Autodesk Fusion 360 part; units mm, degrees
(part 3 of 3)
sketch "Sketch3" plane through (0, 0, 2) normal (0, 0, 1) x (-1, 0, 0)
  line L0 (-24.5, 34.5) -> (-24.5, 36.0424)
  line L1 (-24.5, 36.0424) -> (-65.0462, 36.0424)
  arc A0 (-65.0462, 36.0424) -> (-67.0462, 34.0424) centre (-65.0462, 34.0424) ccw
  line L2 (-67.0462, 34.0424) -> (-67.0462, -34)
  arc A1 (-67.0462, -34) -> (-65.0462, -36) centre (-65.0462, -34) ccw
  line L3 (-65.0462, -36) -> (72.8538, -36)
  arc A2 (72.8538, -36) -> (74.8538, -34) centre (72.8538, -34) ccw
  line L4 (74.8538, -34) -> (74.8538, 39.752)
  line L5 (74.8538, 39.752) -> (59.4057, 65.8207)
  arc A3 (59.4057, 65.8207) -> (56.6719, 66.5254) centre (57.6851, 64.8011) ccw
  line L6 (56.6719, 66.5254) -> (39.1, 56.2)
  line L7 (39.1, 56.2) -> (21.4538, 51.2983)
  line L8 (21.4538, 51.2983) -> (1.5, 51.2983)
  arc A4 (1.5, 51.2983) -> (-0.5, 49.2983) centre (1.5, 49.2983) ccw
  line L9 (-0.5, 49.2983) -> (-0.5, 34.5)
  arc A5 (-2.5, 32.5) -> (-0.5, 34.5) centre (-2.5, 34.5) ccw
  line L10 (-2.5, 32.5) -> (-22.5, 32.5)
  arc A6 (-24.5, 34.5) -> (-22.5, 32.5) centre (-22.5, 34.5) ccw
  circle A7 centre (65.4538, 25.6424) radius 1.5875
  circle A8 centre (-60.5462, -28.3576) radius 1.5875
  circle A9 centre (65.4538, 25.6424) radius 2.45
  circle A10 centre (65.4538, 25.6424) radius 3.45
  circle A11 centre (-60.5462, -28.3576) radius 2.45
  circle A12 centre (-60.5462, -28.3576) radius 3.45
  point P0 (-60.5462, -28.3576)
  dimension "d14" = 4.9
  dimension "d15" = 1
  dimension "d16" = 4.9
  dimension "d17" = 1
  constraint concentric A7 A9
  constraint coincident P0 A8.centre
  measures "d14" diameter of A9
  measures "d16" diameter of A11
extrude "Extrude5" add sketch "Sketch3" along normal blind 4.9 contours A10 | A12
sketch "swopeniing" plane through (-81.8538, 0, 0) normal (-1, 0, 0) x (0, -1, 0)
  line L0 (-40, 0) -> (41.6703, 0)
  line L1 (41.6703, 10.5) -> (-40, 10.5)
  line L2 (-40, 10.5) -> (-40, 0)
  line L3 (41.6703, 0) -> (41.6703, 10.5)
  line L4 (18.0355, 9.995) -> (18.1755, 9.995)
  arc A0 (13.3155, 9.995) -> (13.6755, 10.355) centre (13.3155, 10.355) ccw
  line L5 (11.8255, 9.995) -> (13.1755, 9.995)
  line L6 (17.6755, 12.195) -> (17.6755, 10.355)
  line L7 (18.1755, 9.995) -> (19.5255, 9.995)
  line L8 (13.6755, 10.355) -> (13.6755, 12.195)
  line L9 (19.5255, 12.895) -> (11.8255, 12.895)
  line L10 (13.6755, 12.195) -> (17.6755, 12.195)
  arc A1 (17.6755, 10.355) -> (18.0355, 9.995) centre (18.0355, 10.355) ccw
  line L11 (11.8255, 12.895) -> (11.8255, 9.995)
  line L12 (19.5255, 9.995) -> (19.5255, 12.895)
  line L13 (13.1755, 9.995) -> (13.3155, 9.995)
  line L14 (18.1255, 9.995) -> (13.2255, 9.995)
extrude "Extrude6" cut sketch "swopeniing" against normal blind 20 contours L1 A0 L5 L8 L11 L13 L14 | L1 L4 L6 L7 A1 L12 L14 | L1 A0 L6 L8 A1 L14
sketch "Niceusbopeninig2" plane through (0, 43, 0) normal (0, 1, 0) x (-1, 0, 0)
  line L0 (-71.0462, 0) -> (78.8538, 0)
  line L1 (-71.0462, 10.5) -> (-71.0462, 0)
  line L2 (78.8538, 10.5) -> (-71.0462, 10.5)
  line L3 (78.8538, 0) -> (78.8538, 10.5)
  line L4 (68.0221, 12.5789) -> (68.2393, 12.4584)
  line L5 (68.2393, 12.4584) -> (68.4202, 12.3136)
  line L6 (68.0221, 9.6111) -> (67.7927, 9.5384)
  line L7 (68.7819, 11.4327) -> (68.7819, 10.7693)
  line L8 (68.4202, 12.3136) -> (68.577, 12.1207)
  line L9 (67.7927, 9.5384) -> (67.5393, 9.5145)
  line L10 (68.7579, 11.6741) -> (68.7819, 11.4327)
  line L11 (67.5393, 9.5145) -> (61.085, 9.5145)
  line L12 (59.8424, 11.4327) -> (59.8664, 11.6741)
  line L13 (60.0473, 10.0696) -> (59.9388, 10.2745)
  line L14 (59.9388, 10.2745) -> (59.8664, 10.5159)
  line L15 (60.3853, 9.7316) -> (60.2041, 9.8767)
  line L16 (60.2041, 9.8767) -> (60.0473, 10.0696)
  line L17 (59.8664, 10.5159) -> (59.8424, 10.7693)
  line L18 (59.8424, 10.7693) -> (59.8424, 11.4327)
  line L19 (59.9388, 11.9152) -> (60.0473, 12.1207)
  line L20 (60.2041, 12.3136) -> (60.3853, 12.4584)
  line L21 (67.5393, 12.6755) -> (67.7927, 12.6513)
  line L22 (61.085, 12.6755) -> (67.5393, 12.6755)
  line L23 (60.3853, 12.4584) -> (60.6025, 12.5789)
  line L24 (67.7927, 12.6513) -> (68.0221, 12.5789)
  line L25 (60.6025, 9.6111) -> (60.3853, 9.7316)
  line L26 (68.2393, 9.7316) -> (68.0221, 9.6111)
  line L27 (61.085, 9.5145) -> (60.8316, 9.5384)
  line L28 (60.6025, 12.5789) -> (60.8316, 12.6513)
  line L29 (60.0473, 12.1207) -> (60.2041, 12.3136)
  line L30 (60.8316, 9.5384) -> (60.6025, 9.6111)
  line L31 (68.6853, 10.2745) -> (68.577, 10.0696)
  line L32 (59.8664, 11.6741) -> (59.9388, 11.9152)
  line L33 (68.6853, 11.9152) -> (68.7579, 11.6741)
  line L34 (68.4202, 9.8767) -> (68.2393, 9.7316)
  line L35 (60.8316, 12.6513) -> (61.085, 12.6755)
  line L36 (68.7819, 10.7693) -> (68.7579, 10.5159)
  line L37 (68.577, 10.0696) -> (68.4202, 9.8767)
  line L38 (68.577, 12.1207) -> (68.6853, 11.9152)
  line L39 (68.7579, 10.5159) -> (68.6853, 10.2745)
extrude "Extrude7" cut sketch "Niceusbopeninig2" against normal blind 68 contours L2 L6 L9 L11 L13 L14 L15 L16 L25 L26 L27 L30 L31 L34 L37 L39
